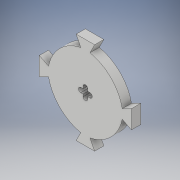
# Autodesk Inventor part: SpinBlade1
Saved by Autodesk Inventor 2017 (Build 210142000, 142)
## iProperties
Created: 2016-10-28
Part Number: SpinBlade1
Material: Generic
Document SubType Name: Modeling
Designer: JJ
Density: 1 g/cm^3
Appearance: Default
Author: JJ
Autodesk Inventor part; units mm, degrees
ref_plane "YZ Plane" through (0, 0, 0) normal (1, 0, 0) x (0, 1, 0)
ref_plane "XZ Plane" through (0, 0, 0) normal (0, 1, 0) x (-1, 0, 0)
ref_plane "XY Plane" through (0, 0, 0) normal (0, 0, 1) x (1, 0, 0)
sketch "Sketch1" plane through (0, 0, 0) normal (0, 0, 1) x (1, 0, 0)
  line L0 (0, 0) -> (0, 50)
  line L1 (0, 0) -> (50, 0)
  line L2 (0, 0) -> (-50, 0)
  line L3 (0, 0) -> (0, -50)
  line L4 (0, 0) -> (5, 0)
  line L5 (0, 0) -> (0, -5)
  line L6 (0, 0) -> (-5, 0)
  line L7 (0, 0) -> (0, 5)
  line L8 (0, -5) -> (40, -5)
  line L9 (0, 5) -> (40, 5)
  line L10 (5, 0) -> (5, 40)
  line L11 (-5, 0) -> (-5, 40)
  line L12 (0, 5) -> (-40, 5)
  line L13 (0, -5) -> (-40, -5)
  line L14 (-5, 0) -> (-5, -40)
  line L15 (5, 0) -> (5, -40)
  arc A0 (-5, 40) -> (-40, 5) centre (4.0754, -4.0754) ccw
  arc A1 (40, 5) -> (5, 40) centre (-4.0754, -4.0754) ccw
  arc A2 (5, -40) -> (40, -5) centre (-4.0754, 4.0754) ccw
  arc A3 (-40, -5) -> (-5, -40) centre (4.0754, 4.0754) ccw
  line L16 (-5, 40) -> (-5, 50)
  line L17 (5, 40) -> (5, 50)
  line L18 (40, 5) -> (50, 5)
  line L19 (40, -5) -> (50, -5)
  line L20 (-5, -40) -> (-5, -50)
  line L21 (5, -40) -> (5, -50)
  line L22 (-40, -5) -> (-50, -5)
  line L23 (-40, 5) -> (-50, 5)
  line L24 (-5, 50) -> (-10, 50)
  line L25 (-10, 50) -> (10, 50)
  line L26 (50, 5) -> (50, 10)
  line L27 (50, 10) -> (50, -10)
  line L28 (5, -50) -> (10, -50)
  line L29 (10, -50) -> (-10, -50)
  line L30 (-50, -5) -> (-50, -10)
  line L31 (-50, -10) -> (-50, 10)
  line L32 (10, 50) -> (5, 40)
  line L33 (-10, 50) -> (-5, 40)
  line L34 (-50, 10) -> (-40, 5)
  line L35 (-50, -10) -> (-40, -5)
  line L36 (-10, -50) -> (-5, -40)
  line L37 (5, -40) -> (10, -50)
  line L38 (40, -5) -> (50, -10)
  line L39 (50, 10) -> (40, 5)
  dimension "d4" = 5
  dimension "d5" = 5
  dimension "d6" = 5
  dimension "d7" = 5
  dimension "d17" = 45
  dimension "d18" = 45
  dimension "d19" = 45
  dimension "d20" = 45
  dimension "d22" = 10
  dimension "d23" = 10
  dimension "d24" = 10
  dimension "d25" = 10
  dimension "d26" = 10
  dimension "d27" = 10
  dimension "d36" = 5
  dimension "d37" = 20
  dimension "d38" = 5
  dimension "d39" = 20
  dimension "d40" = 5
  dimension "d41" = 20
  dimension "d42" = 5
  dimension "d43" = 20
  constraints: 80 end point, 9 horizontal, 9 vertical, 8 point on circle, 8 point on line, 7 perpendicular, 4 centre point, 2 parallel
  measures "d4" distance of L0.start L4.end
  measures "d5" distance of L0.start L5.end
  measures "d6" distance of L0.start L6.end
  measures "d7" distance of L0.start L7.end
  measures "d17" radius of A0
  measures "d18" radius of A1
  measures "d19" radius of A2
  measures "d20" radius of A3
  measures "d22" distance of L11.end L16.end
  measures "d23" distance of L10.end L17.end
  measures "d24" distance of L9.end L18.end
  measures "d25" distance of L14.end L20.end
  measures "d26" distance of L13.end L22.end
  measures "d27" distance of L12.end L23.end
  measures "d36" distance of L16.end L24.end
  measures "d37" distance of L24.end L25.end
  measures "d38" distance of L18.end L26.end
  measures "d39" distance of L26.end L27.end
  measures "d40" distance of L21.end L28.end
  measures "d41" distance of L28.end L29.end
  measures "d42" distance of L22.end L30.end
  measures "d43" distance of L30.end L31.end
extrude "Extrusion3" add sketch "Sketch1" along normal blind 10
sketch "Sketch3" plane through (0, 0, 10) normal (0, 0, 1) x (1, 0, 0)
  line L0 (0, -5) -> (0, 5) construction
  line L1 (2.5, -5) -> (2.5, 5)
  line L2 (-2.5, 5) -> (-2.5, -5)
  arc A0 (-2.5, -5) -> (2.5, -5) centre (0, -5) ccw
  arc A1 (2.5, 5) -> (-2.5, 5) centre (0, 5) ccw
  line L3 (5, 0) -> (-5, 0) construction
  line L4 (5, 2.5) -> (-5, 2.5)
  line L5 (-5, -2.5) -> (5, -2.5)
  arc A2 (5, -2.5) -> (5, 2.5) centre (5, 0) ccw
  arc A3 (-5, 2.5) -> (-5, -2.5) centre (-5, 0) ccw
  point P0 (0, 0)
  dimension "d47" = 5
  dimension "d48" = 5
  dimension "d49" = 5
  dimension "d50" = 5
  constraints: 16 end point, 8 point on circle, 8 tangent, 4 centre point, 2 midpoint, 2 parallel, 1 horizontal, 1 vertical
  measures "d47" distance of point (0, 0) L0.end
  measures "d48" diameter of A1
  measures "d49" distance of point (0, 0) L3.end
  measures "d50" diameter of A3
extrude "Extrusion4" cut sketch "Sketch3" against normal blind 10
body "Solid2"
